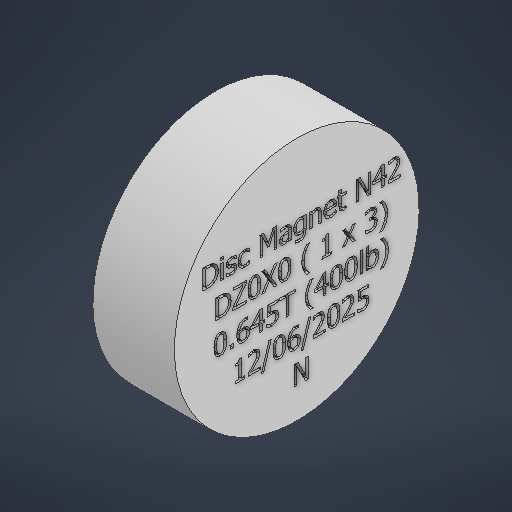
# Autodesk Inventor part: SampleMagnet
Saved by Autodesk Inventor 2026.1 (Build 301233000, 233)
## iProperties
Created: 2025-12-08
Part Number: SampleMagnet
Material: Generic
Document SubType Name: Modeling
Designer: usman
Density: 1 g/cm^3
Appearance: Default
Author: usman
Autodesk Inventor part; units mm, degrees
(part 1 of 2)
ref_plane "YZ Plane" through (0, 0, 0) normal (1, 0, 0) x (0, 1, 0)
ref_plane "XZ Plane" through (0, 0, 0) normal (0, 1, 0) x (-1, 0, 0)
ref_plane "XY Plane" through (0, 0, 0) normal (0, 0, 1) x (1, 0, 0)
sketch "Sketch1" plane through (0, 0, 0) normal (1, 0, 0) x (0, 1, 0)
  circle A0 centre (0, 0) radius 38.1
  dimension "d0" = 76.2
  constraints: 1 centre point, 1 coincident
  measures "d0" diameter of A0
extrude "Extrusion1" add sketch "Sketch1" along normal blind 25.4
sketch "Sketch2" plane through (25.4, 0, 0) normal (1, 0, 0) x (0, 0, -1)
  line L0 (-30.9138, 17.7652) -> (33.738, 17.7652) construction
  line L1 (33.738, 17.7652) -> (33.738, -46.1132) construction
  line L2 (33.738, -46.1132) -> (-30.9138, -46.1132) construction
  line L3 (-30.9138, -46.1132) -> (-30.9138, 17.7652) construction
  spline S0 degree 2 poles (-24.4539, 14.5839) (-24.4539, 13.749) (-25.1307, 12.4053) (-25.6988, 12.0299) knots 0 0 0 1 2 2 2
  spline S1 degree 2 poles (-25.6988, 12.0299) (-26.1632, 11.7384) (-27.1166, 11.5408) (-27.8576, 11.5408) knots 0 0 0 1 2 2 2
  line L4 (-27.8576, 11.5408) -> (-29.2606, 11.5408)
  line L5 (-29.2606, 11.5408) -> (-29.2606, 17.6368)
  line L6 (-29.2606, 17.6368) -> (-27.8724, 17.6368)
  spline S2 degree 2 poles (-27.8724, 17.6368) (-27.0129, 17.6368) (-26.0347, 17.3799) (-25.6889, 17.1527) knots 0 0 0 1 2 2 2
  spline S3 degree 2 poles (-25.6889, 17.1527) (-25.1011, 16.7624) (-24.4539, 15.4731) (-24.4539, 14.5839) knots 0 0 0 1 2 2 2
  spline S4 degree 2 poles (-25.2987, 14.5937) (-25.2987, 15.2952) (-25.763, 16.2882) (-26.2225, 16.5698) knots 0 0 0 1 2 2 2
  spline S5 degree 2 poles (-26.2225, 16.5698) (-26.5485, 16.7624) (-27.2846, 16.9353) (-27.8329, 16.9353) knots 0 0 0 1 2 2 2
  line L7 (-27.8329, 16.9353) -> (-28.4504, 16.9353)
  line L8 (-28.4504, 16.9353) -> (-28.4504, 12.2423)
  line L9 (-28.4504, 12.2423) -> (-27.8329, 12.2423)
  spline S6 degree 2 poles (-27.8329, 12.2423) (-27.2945, 12.2423) (-26.4793, 12.4152) (-26.1484, 12.6474) knots 0 0 0 1 2 2 2
  spline S7 degree 2 poles (-26.1484, 12.6474) (-25.7235, 12.9339) (-25.2987, 13.8824) (-25.2987, 14.5937) knots 0 0 0 1 2 2 2
  line L10 (-22.8484, 11.5408) -> (-23.6191, 11.5408)
  line L11 (-23.6191, 11.5408) -> (-23.6191, 16.1153)
  line L12 (-23.6191, 16.1153) -> (-22.8484, 16.1153)
  line L13 (-22.8484, 16.1153) -> (-22.8484, 11.5408)
  line L14 (-22.7941, 16.876) -> (-23.6685, 16.876)
  line L15 (-23.6685, 16.876) -> (-23.6685, 17.6763)
  line L16 (-23.6685, 17.6763) -> (-22.7941, 17.6763)
  line L17 (-22.7941, 17.6763) -> (-22.7941, 16.876)
  spline S8 degree 2 poles (-20.4821, 11.4321) (-20.9416, 11.4321) (-21.7369, 11.6791) (-21.9987, 11.8174) knots 0 0 0 1 2 2 2
  line L18 (-21.9987, 11.8174) -> (-21.9987, 12.6819)
  line L19 (-21.9987, 12.6819) -> (-21.9592, 12.6819)
  spline S9 degree 2 poles (-21.9592, 12.6819) (-21.8604, 12.6029) (-21.5937, 12.4152) (-21.3714, 12.3114) knots 0 0 0 1 2 2 2
  spline S10 degree 2 poles (-21.3714, 12.3114) (-21.1787, 12.2176) (-20.7044, 12.0793) (-20.4525, 12.0793) knots 0 0 0 1 2 2 2
  spline S11 degree 2 poles (-20.4525, 12.0793) (-20.2697, 12.0793) (-19.8498, 12.1632) (-19.751, 12.2324) knots 0 0 0 1 2 2 2
  spline S12 degree 2 poles (-19.751, 12.2324) (-19.6078, 12.3263) (-19.4793, 12.5387) (-19.4793, 12.756) knots 0 0 0 1 2 2 2
  spline S13 degree 2 poles (-19.4793, 12.756) (-19.4793, 13.0278) (-19.7757, 13.3093) (-20.1561, 13.4032) knots 0 0 0 1 2 2 2
  spline S14 degree 2 poles (-20.1561, 13.4032) (-20.3043, 13.4378) (-20.7786, 13.5366) (-20.9811, 13.5909) knots 0 0 0 1 2 2 2
  spline S15 degree 2 poles (-20.9811, 13.5909) (-21.5047, 13.7441) (-21.979, 14.3764) (-21.979, 14.8259) knots 0 0 0 1 2 2 2
  spline S16 degree 2 poles (-21.979, 14.8259) (-21.979, 15.4484) (-21.0453, 16.224) (-20.2747, 16.224) knots 0 0 0 1 2 2 2
  spline S17 degree 2 poles (-20.2747, 16.224) (-19.8943, 16.224) (-19.1236, 16.0362) (-18.8618, 15.893) knots 0 0 0 1 2 2 2
  line L20 (-18.8618, 15.893) -> (-18.8618, 15.068)
  line L21 (-18.8618, 15.068) -> (-18.9013, 15.068)
  spline S18 degree 2 poles (-18.9013, 15.068) (-19.1977, 15.3051) (-19.919, 15.5768) (-20.2895, 15.5768) knots 0 0 0 1 2 2 2
  spline S19 degree 2 poles (-20.2895, 15.5768) (-20.6699, 15.5768) (-21.1935, 15.2557) (-21.1935, 14.9346) knots 0 0 0 1 2 2 2
  spline S20 degree 2 poles (-21.1935, 14.9346) (-21.1935, 14.6431) (-20.8823, 14.3616) (-20.5365, 14.2726) knots 0 0 0 1 2 2 2
  spline S21 degree 2 poles (-20.5365, 14.2726) (-20.3685, 14.2282) (-19.9437, 14.1393) (-19.7115, 14.0849) knots 0 0 0 1 2 2 2
  spline S22 degree 2 poles (-19.7115, 14.0849) (-19.2076, 13.9565) (-18.6939, 13.3686) (-18.6939, 12.8598) knots 0 0 0 1 2 2 2
  spline S23 degree 2 poles (-18.6939, 12.8598) (-18.6939, 12.5634) (-18.926, 12.0397) (-19.1533, 11.8471) knots 0 0 0 1 2 2 2
  spline S24 degree 2 poles (-19.1533, 11.8471) (-19.3953, 11.6445) (-20.0128, 11.4321) (-20.4821, 11.4321) knots 0 0 0 1 2 2 2
  spline S25 degree 2 poles (-16.1596, 11.4371) (-16.6339, 11.4371) (-17.4193, 11.7285) (-17.7009, 12.0249) knots 0 0 0 1 2 2 2
  spline S26 degree 2 poles (-17.7009, 12.0249) (-17.9825, 12.3164) (-18.2937, 13.2155) (-18.2937, 13.8182) knots 0 0 0 1 2 2 2
  spline S27 degree 2 poles (-18.2937, 13.8182) (-18.2937, 14.4208) (-17.9726, 15.3002) (-17.7009, 15.5966) knots 0 0 0 1 2 2 2
  spline S28 degree 2 poles (-17.7009, 15.5966) (-17.4292, 15.8979) (-16.624, 16.219) (-16.1596, 16.219) knots 0 0 0 1 2 2 2
  spline S29 degree 2 poles (-16.1596, 16.219) (-15.7842, 16.219) (-15.0827, 16.0066) (-14.811, 15.8683) knots 0 0 0 1 2 2 2
  line L22 (-14.811, 15.8683) -> (-14.811, 15.0038)
  line L23 (-14.811, 15.0038) -> (-14.8555, 15.0038)
  spline S30 degree 2 poles (-14.8555, 15.0038) (-14.9394, 15.0729) (-15.1963, 15.2508) (-15.3791, 15.3446) knots 0 0 0 1 2 2 2
  spline S31 degree 2 poles (-15.3791, 15.3446) (-15.5421, 15.4237) (-15.9768, 15.5472) (-16.1744, 15.5472) knots 0 0 0 1 2 2 2
  spline S32 degree 2 poles (-16.1744, 15.5472) (-16.7722, 15.5472) (-17.4984, 14.6431) (-17.4984, 13.8182) knots 0 0 0 1 2 2 2
  spline S33 degree 2 poles (-17.4984, 13.8182) (-17.4984, 13.0129) (-16.7969, 12.1089) (-16.1744, 12.1089) knots 0 0 0 1 2 2 2
  spline S34 degree 2 poles (-16.1744, 12.1089) (-15.799, 12.1089) (-15.1173, 12.4201) (-14.8555, 12.6622) knots 0 0 0 1 2 2 2
  line L24 (-14.8555, 12.6622) -> (-14.811, 12.6622)
  line L25 (-14.811, 12.6622) -> (-14.811, 11.7977)
  spline S35 degree 2 poles (-14.811, 11.7977) (-14.9246, 11.7433) (-15.2704, 11.5902) (-15.4087, 11.5556) knots 0 0 0 1 2 2 2
  spline S36 degree 2 poles (-15.4087, 11.5556) (-15.6063, 11.4963) (-15.9176, 11.4371) (-16.1596, 11.4371) knots 0 0 0 1 2 2 2
  line L26 (-6.2055, 11.5408) -> (-7.0156, 11.5408)
  line L27 (-7.0156, 11.5408) -> (-7.0156, 16.7921)
  line L28 (-7.0156, 16.7921) -> (-8.6063, 13.2204)
  line L29 (-8.6063, 13.2204) -> (-9.1003, 13.2204)
  line L30 (-9.1003, 13.2204) -> (-10.6762, 16.7921)
  line L31 (-10.6762, 16.7921) -> (-10.6762, 11.5408)
  line L32 (-10.6762, 11.5408) -> (-11.432, 11.5408)
  line L33 (-11.432, 11.5408) -> (-11.432, 17.6368)
  line L34 (-11.432, 17.6368) -> (-10.3254, 17.6368)
  line L35 (-10.3254, 17.6368) -> (-8.8039, 14.243)
  line L36 (-8.8039, 14.243) -> (-7.3318, 17.6368)
  line L37 (-7.3318, 17.6368) -> (-6.2055, 17.6368)
  line L38 (-6.2055, 17.6368) -> (-6.2055, 11.5408)
  spline S37 degree 2 poles (-2.4807, 12.0249) (-2.5745, 11.9558) (-2.8907, 11.7088) (-3.0389, 11.6347) knots 0 0 0 1 2 2 2
  spline S38 degree 2 poles (-3.0389, 11.6347) (-3.2414, 11.526) (-3.6218, 11.4124) (-3.9676, 11.4124) knots 0 0 0 1 2 2 2
  spline S39 degree 2 poles (-3.9676, 11.4124) (-4.2492, 11.4124) (-4.758, 11.6248) (-4.9507, 11.8174) knots 0 0 0 1 2 2 2
  spline S40 degree 2 poles (-4.9507, 11.8174) (-5.1335, 12.0052) (-5.3558, 12.5584) (-5.3558, 12.8647) knots 0 0 0 1 2 2 2
  spline S41 degree 2 poles (-5.3558, 12.8647) (-5.3558, 13.339) (-4.9556, 14.0108) (-4.5209, 14.2035) knots 0 0 0 1 2 2 2
  spline S42 degree 2 poles (-4.5209, 14.2035) (-4.1356, 14.3813) (-3.0883, 14.5147) (-2.4807, 14.5493) knots 0 0 0 1 2 2 2
  line L39 (-2.4807, 14.5493) -> (-2.4807, 14.6975)
  spline S43 degree 2 poles (-2.4807, 14.6975) (-2.4807, 14.9642) (-2.6437, 15.2952) (-2.7919, 15.3891) knots 0 0 0 1 2 2 2
  spline S44 degree 2 poles (-2.7919, 15.3891) (-2.9401, 15.4829) (-3.3649, 15.5422) (-3.5922, 15.5422) knots 0 0 0 1 2 2 2
  spline S45 degree 2 poles (-3.5922, 15.5422) (-3.8589, 15.5422) (-4.5802, 15.3841) (-4.9408, 15.231) knots 0 0 0 1 2 2 2
  line L40 (-4.9408, 15.231) -> (-4.9853, 15.231)
  line L41 (-4.9853, 15.231) -> (-4.9853, 16.0165)
  spline S46 degree 2 poles (-4.9853, 16.0165) (-4.7728, 16.0758) (-3.9775, 16.224) (-3.5872, 16.224) knots 0 0 0 1 2 2 2
  spline S47 degree 2 poles (-3.5872, 16.224) (-3.113, 16.224) (-2.4658, 16.0758) (-2.209, 15.8831) knots 0 0 0 1 2 2 2
  spline S48 degree 2 poles (-2.209, 15.8831) (-1.957, 15.6954) (-1.71, 15.0976) (-1.71, 14.6678) knots 0 0 0 1 2 2 2
  line L42 (-1.71, 14.6678) -> (-1.71, 11.5408)
  line L43 (-1.71, 11.5408) -> (-2.4807, 11.5408)
  line L44 (-2.4807, 11.5408) -> (-2.4807, 12.0249)
  line L45 (-2.4807, 12.6671) -> (-2.4807, 13.9367)
  spline S49 degree 2 poles (-2.4807, 13.9367) (-2.7573, 13.912) (-3.5922, 13.828) (-3.854, 13.749) knots 0 0 0 1 2 2 2
  spline S50 degree 2 poles (-3.854, 13.749) (-4.1603, 13.6551) (-4.5604, 13.2649) (-4.5604, 12.9191) knots 0 0 0 1 2 2 2
  spline S51 degree 2 poles (-4.5604, 12.9191) (-4.5604, 12.5239) (-4.1158, 12.1237) (-3.691, 12.1237) knots 0 0 0 1 2 2 2
  spline S52 degree 2 poles (-3.691, 12.1237) (-3.3304, 12.1237) (-2.7376, 12.4349) (-2.4807, 12.6671) knots 0 0 0 1 2 2 2
  spline S53 degree 2 poles (-0.4651, 10.8097) (-0.3861, 10.7751) (-0.0848, 10.6664) (0.1079, 10.622) knots 0 0 0 1 2 2 2
  spline S54 degree 2 poles (0.1079, 10.622) (0.3203, 10.5676) (0.681, 10.5034) (0.8934, 10.5034) knots 0 0 0 1 2 2 2
  spline S55 degree 2 poles (0.8934, 10.5034) (1.2491, 10.5034) (1.7431, 10.6911) (1.8814, 10.8591) knots 0 0 0 1 2 2 2
  spline S56 degree 2 poles (1.8814, 10.8591) (2.0148, 11.027) (2.1185, 11.4667) (2.1185, 11.7483) knots 0 0 0 1 2 2 2
  line L46 (2.1185, 11.7483) -> (2.1185, 12.1484)
  spline S57 degree 2 poles (2.1185, 12.1484) (1.8073, 11.8767) (1.2095, 11.6198) (0.76, 11.6198) knots 0 0 0 1 2 2 2
  spline S58 degree 2 poles (0.76, 11.6198) (-0.0205, 11.6198) (-0.9443, 12.7807) (-0.9443, 13.8725) knots 0 0 0 1 2 2 2
  spline S59 degree 2 poles (-0.9443, 13.8725) (-0.9443, 14.4406) (-0.6232, 15.3199) (-0.3565, 15.6311) knots 0 0 0 1 2 2 2
  spline S60 degree 2 poles (-0.3565, 15.6311) (-0.0996, 15.9226) (0.6069, 16.2437) (0.9823, 16.2437) knots 0 0 0 1 2 2 2
  spline S61 degree 2 poles (0.9823, 16.2437) (1.338, 16.2437) (1.8567, 16.0758) (2.1185, 15.9226) knots 0 0 0 1 2 2 2
  line L47 (2.1185, 15.9226) -> (2.163, 16.1153)
  line L48 (2.163, 16.1153) -> (2.8891, 16.1153)
  line L49 (2.8891, 16.1153) -> (2.8891, 12.0644)
  spline S62 degree 2 poles (2.8891, 12.0644) (2.8891, 10.8986) (1.8764, 9.8118) (0.8341, 9.8118) knots 0 0 0 1 2 2 2
  spline S63 degree 2 poles (0.8341, 9.8118) (0.4982, 9.8118) (-0.2033, 9.9205) (-0.5047, 10.0094) knots 0 0 0 1 2 2 2
  line L50 (-0.5047, 10.0094) -> (-0.5047, 10.8097)
  line L51 (-0.5047, 10.8097) -> (-0.4651, 10.8097)
  line L52 (2.1185, 12.7807) -> (2.1185, 15.2952)
  spline S64 degree 2 poles (2.1185, 15.2952) (1.832, 15.4335) (1.3479, 15.5521) (1.1058, 15.5521) knots 0 0 0 1 2 2 2
  spline S65 degree 2 poles (1.1058, 15.5521) (0.5229, 15.5521) (-0.149, 14.6925) (-0.149, 13.8873) knots 0 0 0 1 2 2 2
  spline S66 degree 2 poles (-0.149, 13.8873) (-0.149, 13.1266) (0.3598, 12.3312) (0.9329, 12.3312) knots 0 0 0 1 2 2 2
  spline S67 degree 2 poles (0.9329, 12.3312) (1.2342, 12.3312) (1.8666, 12.5683) (2.1185, 12.7807) knots 0 0 0 1 2 2 2
  line L53 (7.597, 11.5408) -> (6.8264, 11.5408)
  line L54 (6.8264, 11.5408) -> (6.8264, 14.1491)
  spline S68 degree 2 poles (6.8264, 14.1491) (6.8264, 14.4653) (6.7671, 15.0087) (6.6782, 15.1717) knots 0 0 0 1 2 2 2
  spline S69 degree 2 poles (6.6782, 15.1717) (6.5843, 15.3446) (6.2484, 15.5126) (5.9618, 15.5126) knots 0 0 0 1 2 2 2
  spline S70 degree 2 poles (5.9618, 15.5126) (5.6753, 15.5126) (5.0677, 15.2063) (4.7762, 14.9593) knots 0 0 0 1 2 2 2
  line L55 (4.7762, 14.9593) -> (4.7762, 11.5408)
  line L56 (4.7762, 11.5408) -> (4.0056, 11.5408)
  line L57 (4.0056, 11.5408) -> (4.0056, 16.1153)
  line L58 (4.0056, 16.1153) -> (4.7762, 16.1153)
  line L59 (4.7762, 16.1153) -> (4.7762, 15.6064)
  spline S71 degree 2 poles (4.7762, 15.6064) (5.122, 15.9177) (5.7889, 16.2437) (6.1644, 16.2437) knots 0 0 0 1 2 2 2
  spline S72 degree 2 poles (6.1644, 16.2437) (6.8362, 16.2437) (7.597, 15.3545) (7.597, 14.5098) knots 0 0 0 1 2 2 2
  line L60 (7.597, 14.5098) -> (7.597, 11.5408)
  spline S73 degree 2 poles (10.6648, 11.4371) (9.5681, 11.4371) (8.3627, 12.6671) (8.3627, 13.8033) knots 0 0 0 1 2 2 2
  spline S74 degree 2 poles (8.3627, 13.8033) (8.3627, 14.9198) (9.5335, 16.2437) (10.477, 16.2437) knots 0 0 0 1 2 2 2
  spline S75 degree 2 poles (10.477, 16.2437) (10.9019, 16.2437) (11.5589, 15.9967) (11.801, 15.7349) knots 0 0 0 1 2 2 2
  spline S76 degree 2 poles (11.801, 15.7349) (12.048, 15.4731) (12.3098, 14.7172) (12.3098, 14.1689) knots 0 0 0 1 2 2 2
  line L61 (12.3098, 14.1689) -> (12.3098, 13.749)
  line L62 (12.3098, 13.749) -> (9.1432, 13.749)
  spline S77 degree 2 poles (9.1432, 13.749) (9.1432, 12.9537) (9.9435, 12.1089) (10.6549, 12.1089) knots 0 0 0 1 2 2 2
  spline S78 degree 2 poles (10.6549, 12.1089) (10.9068, 12.1089) (11.3959, 12.2225) (11.5935, 12.3114) knots 0 0 0 1 2 2 2
  spline S79 degree 2 poles (11.5935, 12.3114) (11.801, 12.4102) (12.0875, 12.5831) (12.1813, 12.6622) knots 0 0 0 1 2 2 2
  line L63 (12.1813, 12.6622) -> (12.2258, 12.6622)
  line L64 (12.2258, 12.6622) -> (12.2258, 11.8224)
  spline S80 degree 2 poles (12.2258, 11.8224) (12.0924, 11.768) (11.6873, 11.61) (11.5293, 11.5655) knots 0 0 0 1 2 2 2
  spline S81 degree 2 poles (11.5293, 11.5655) (11.307, 11.5013) (10.9414, 11.4371) (10.6648, 11.4371) knots 0 0 0 1 2 2 2
  spline S82 degree 2 poles (11.5589, 14.3369) (11.549, 14.6481) (11.4206, 15.1026) (11.2971, 15.2557) knots 0 0 0 1 2 2 2
  spline S83 degree 2 poles (11.2971, 15.2557) (11.1637, 15.4286) (10.7438, 15.6114) (10.4326, 15.6114) knots 0 0 0 1 2 2 2
  spline S84 degree 2 poles (10.4326, 15.6114) (10.1263, 15.6114) (9.6965, 15.4286) (9.5187, 15.2508) knots 0 0 0 1 2 2 2
  spline S85 degree 2 poles (9.5187, 15.2508) (9.3458, 15.068) (9.1679, 14.6283) (9.1432, 14.3369) knots 0 0 0 1 2 2 2
  line L65 (9.1432, 14.3369) -> (11.5589, 14.3369)
  spline S86 degree 2 poles (14.4735, 11.4519) (13.8461, 11.4519) (13.1397, 12.1682) (13.1397, 12.9438) knots 0 0 0 1 2 2 2
  line L66 (13.1397, 12.9438) -> (13.1397, 15.478)
  line L67 (13.1397, 15.478) -> (12.621, 15.478)
  line L68 (12.621, 15.478) -> (12.621, 16.1153)
  line L69 (12.621, 16.1153) -> (13.1397, 16.1153)
  line L70 (13.1397, 16.1153) -> (13.1397, 17.4293)
  line L71 (13.1397, 17.4293) -> (13.9104, 17.4293)
  line L72 (13.9104, 17.4293) -> (13.9104, 16.1153)
  line L73 (13.9104, 16.1153) -> (15.3281, 16.1153)
  line L74 (15.3281, 16.1153) -> (15.3281, 15.478)
  line L75 (15.3281, 15.478) -> (13.9104, 15.478)
  line L76 (13.9104, 15.478) -> (13.9104, 13.2995)
  spline S87 degree 2 poles (13.9104, 13.2995) (13.9104, 12.9537) (13.9351, 12.5733) (14.019, 12.4102) knots 0 0 0 1 2 2 2
  spline S88 degree 2 poles (14.019, 12.4102) (14.0882, 12.267) (14.3994, 12.1237) (14.6662, 12.1237) knots 0 0 0 1 2 2 2
  spline S89 degree 2 poles (14.6662, 12.1237) (14.8539, 12.1237) (15.2046, 12.2373) (15.2837, 12.2719) knots 0 0 0 1 2 2 2
  line L77 (15.2837, 12.2719) -> (15.3281, 12.2719)
  line L78 (15.3281, 12.2719) -> (15.3281, 11.5803)
  spline S90 degree 2 poles (15.3281, 11.5803) (15.1108, 11.521) (14.6662, 11.4519) (14.4735, 11.4519) knots 0 0 0 1 2 2 2
  line L79 (22.9358, 11.5408) -> (22.0268, 11.5408)
  line L80 (22.0268, 11.5408) -> (19.3296, 16.797)
  line L81 (19.3296, 16.797) -> (19.3296, 11.5408)
  line L82 (19.3296, 11.5408) -> (18.5737, 11.5408)
  line L83 (18.5737, 11.5408) -> (18.5737, 17.6368)
  line L84 (18.5737, 17.6368) -> (19.7248, 17.6368)
  line L85 (19.7248, 17.6368) -> (22.18, 12.8104)
  line L86 (22.18, 12.8104) -> (22.18, 17.6368)
  line L87 (22.18, 17.6368) -> (22.9358, 17.6368)
  line L88 (22.9358, 17.6368) -> (22.9358, 11.5408)
  line L89 (27.9203, 13.6354) -> (27.1941, 13.6354)
  line L90 (27.1941, 13.6354) -> (27.1941, 11.5408)
  line L91 (27.1941, 11.5408) -> (26.4086, 11.5408)
  line L92 (26.4086, 11.5408) -> (26.4086, 13.6354)
  line L93 (26.4086, 13.6354) -> (23.7163, 13.6354)
  line L94 (23.7163, 13.6354) -> (23.7163, 14.4949)
  line L95 (23.7163, 14.4949) -> (26.4432, 17.6368)
  line L96 (26.4432, 17.6368) -> (27.1941, 17.6368)
  line L97 (27.1941, 17.6368) -> (27.1941, 14.2924)
  line L98 (27.1941, 14.2924) -> (27.9203, 14.2924)
  line L99 (27.9203, 14.2924) -> (27.9203, 13.6354)
  line L100 (26.4086, 14.2924) -> (26.4086, 16.6735)
  line L101 (26.4086, 16.6735) -> (24.3585, 14.2924)
  line L102 (24.3585, 14.2924) -> (26.4086, 14.2924)
  line L103 (32.3317, 11.5408) -> (28.5724, 11.5408)
  line L104 (28.5724, 11.5408) -> (28.5724, 12.4053)
  spline S91 degree 2 poles (28.5724, 12.4053) (28.9775, 12.7857) (29.6987, 13.4921) (30.0445, 13.8725) knots 0 0 0 1 2 2 2
  spline S92 degree 2 poles (30.0445, 13.8725) (30.741, 14.6382) (31.2499, 15.557) (31.2499, 16.0461) knots 0 0 0 1 2 2 2
  spline S93 degree 2 poles (31.2499, 16.0461) (31.2499, 16.303) (31.0918, 16.6883) (30.9485, 16.8118) knots 0 0 0 1 2 2 2
  spline S94 degree 2 poles (30.9485, 16.8118) (30.8053, 16.9353) (30.4298, 17.0588) (30.2026, 17.0588) knots 0 0 0 1 2 2 2
  spline S95 degree 2 poles (30.2026, 17.0588) (29.9852, 17.0588) (29.5406, 16.9501) (29.3381, 16.8662) knots 0 0 0 1 2 2 2
  spline S96 degree 2 poles (29.3381, 16.8662) (29.1652, 16.797) (28.8441, 16.5994) (28.7453, 16.5302) knots 0 0 0 1 2 2 2
  line L105 (28.7453, 16.5302) -> (28.7008, 16.5302)
  line L106 (28.7008, 16.5302) -> (28.7008, 17.3997)
  spline S97 degree 2 poles (28.7008, 17.3997) (28.9528, 17.5232) (29.8568, 17.7652) (30.2619, 17.7652) knots 0 0 0 1 2 2 2
  spline S98 degree 2 poles (30.2619, 17.7652) (31.1165, 17.7652) (32.0798, 16.8612) (32.0798, 16.0906) knots 0 0 0 1 2 2 2
  spline S99 degree 2 poles (32.0798, 16.0906) (32.0798, 15.7299) (31.9118, 15.1273) (31.7636, 14.8704) knots 0 0 0 1 2 2 2
  spline S100 degree 2 poles (31.7636, 14.8704) (31.6154, 14.6036) (31.1857, 14.08) (30.9485, 13.828) knots 0 0 0 1 2 2 2
  spline S101 degree 2 poles (30.9485, 13.828) (30.5632, 13.4081) (29.6197, 12.509) (29.3381, 12.2472) knots 0 0 0 1 2 2 2
  line L107 (29.3381, 12.2472) -> (32.3317, 12.2472)
  line L108 (32.3317, 12.2472) -> (32.3317, 11.5408)
  spline S102 degree 2 poles (-20.455, 4.547) (-20.455, 3.7121) (-21.1318, 2.3684) (-21.6999, 1.993) knots 0 0 0 1 2 2 2
  spline S103 degree 2 poles (-21.6999, 1.993) (-22.1642, 1.7015) (-23.1177, 1.5039) (-23.8587, 1.5039) knots 0 0 0 1 2 2 2
  line L109 (-23.8587, 1.5039) -> (-25.2616, 1.5039)
  line L110 (-25.2616, 1.5039) -> (-25.2616, 7.5999)
  line L111 (-25.2616, 7.5999) -> (-23.8735, 7.5999)
  spline S104 degree 2 poles (-23.8735, 7.5999) (-23.0139, 7.5999) (-22.0358, 7.343) (-21.69, 7.1158) knots 0 0 0 1 2 2 2
  spline S105 degree 2 poles (-21.69, 7.1158) (-21.1021, 6.7255) (-20.455, 5.4362) (-20.455, 4.547) knots 0 0 0 1 2 2 2
  spline S106 degree 2 poles (-21.2997, 4.5568) (-21.2997, 5.2583) (-21.7641, 6.2513) (-22.2235, 6.5329) knots 0 0 0 1 2 2 2
  spline S107 degree 2 poles (-22.2235, 6.5329) (-22.5496, 6.7255) (-23.2856, 6.8984) (-23.834, 6.8984) knots 0 0 0 1 2 2 2
  line L112 (-23.834, 6.8984) -> (-24.4515, 6.8984)
  line L113 (-24.4515, 6.8984) -> (-24.4515, 2.2054)
  line L114 (-24.4515, 2.2054) -> (-23.834, 2.2054)
  spline S108 degree 2 poles (-23.834, 2.2054) (-23.2955, 2.2054) (-22.4804, 2.3783) (-22.1494, 2.6105) knots 0 0 0 1 2 2 2
  spline S109 degree 2 poles (-22.1494, 2.6105) (-21.7246, 2.897) (-21.2997, 3.8455) (-21.2997, 4.5568) knots 0 0 0 1 2 2 2
  line L115 (-15.6878, 1.5039) -> (-19.9462, 1.5039)
  line L116 (-19.9462, 1.5039) -> (-19.9462, 2.2597)
  line L117 (-19.9462, 2.2597) -> (-16.6857, 6.8787)
  line L118 (-16.6857, 6.8787) -> (-19.798, 6.8787)
  line L119 (-19.798, 6.8787) -> (-19.798, 7.5999)
  line L120 (-19.798, 7.5999) -> (-15.7718, 7.5999)
  line L121 (-15.7718, 7.5999) -> (-15.7718, 6.8688)
  line L122 (-15.7718, 6.8688) -> (-19.0668, 2.2251)
  line L123 (-19.0668, 2.2251) -> (-15.6878, 2.2251)
  line L124 (-15.6878, 2.2251) -> (-15.6878, 1.5039)
  spline S110 degree 2 poles (-11.2665, 4.5519) (-11.2665, 2.9118) (-12.2199, 1.3755) (-13.2129, 1.3755) knots 0 0 0 1 2 2 2
  spline S111 degree 2 poles (-13.2129, 1.3755) (-14.2207, 1.3755) (-15.1642, 2.9414) (-15.1642, 4.547) knots 0 0 0 1 2 2 2
  spline S112 degree 2 poles (-15.1642, 4.547) (-15.1642, 6.1969) (-14.2108, 7.7234) (-13.2129, 7.7234) knots 0 0 0 1 2 2 2
  spline S113 degree 2 poles (-13.2129, 7.7234) (-12.2101, 7.7234) (-11.2665, 6.1426) (-11.2665, 4.5519) knots 0 0 0 1 2 2 2
  spline S114 degree 2 poles (-12.3138, 2.6944) (-12.1952, 2.9958) (-12.0964, 3.9245) (-12.0964, 4.5519) knots 0 0 0 1 2 2 2
  spline S115 degree 2 poles (-12.0964, 4.5519) (-12.0964, 5.1793) (-12.1952, 6.1031) (-12.3187, 6.4143) knots 0 0 0 1 2 2 2
  spline S116 degree 2 poles (-12.3187, 6.4143) (-12.4422, 6.7255) (-12.872, 7.0466) (-13.2129, 7.0466) knots 0 0 0 1 2 2 2
  spline S117 degree 2 poles (-13.2129, 7.0466) (-13.5538, 7.0466) (-13.9934, 6.7255) (-14.1219, 6.4044) knots 0 0 0 1 2 2 2
  spline S118 degree 2 poles (-14.1219, 6.4044) (-14.2454, 6.0932) (-14.3343, 5.1447) (-14.3343, 4.547) knots 0 0 0 1 2 2 2
  spline S119 degree 2 poles (-14.3343, 4.547) (-14.3343, 3.9048) (-14.2552, 3.0452) (-14.1268, 2.7093) knots 0 0 0 1 2 2 2
  spline S120 degree 2 poles (-14.1268, 2.7093) (-14.0082, 2.3931) (-13.5686, 2.0522) (-13.2129, 2.0522) knots 0 0 0 1 2 2 2
  spline S121 degree 2 poles (-13.2129, 2.0522) (-12.877, 2.0522) (-12.4373, 2.3733) (-12.3138, 2.6944) knots 0 0 0 1 2 2 2
  line L125 (-6.0992, 1.5039) -> (-7.028, 1.5039)
  line L126 (-7.028, 1.5039) -> (-8.51, 3.9344)
  line L127 (-8.51, 3.9344) -> (-10.0216, 1.5039)
  line L128 (-10.0216, 1.5039) -> (-10.896, 1.5039)
  line L129 (-10.896, 1.5039) -> (-8.9546, 4.5568)
  line L130 (-8.9546, 4.5568) -> (-10.8367, 7.5999)
  line L131 (-10.8367, 7.5999) -> (-9.908, 7.5999)
  line L132 (-9.908, 7.5999) -> (-8.4556, 5.2139)
  line L133 (-8.4556, 5.2139) -> (-6.9736, 7.5999)
  line L134 (-6.9736, 7.5999) -> (-6.0992, 7.5999)
  line L135 (-6.0992, 7.5999) -> (-8.0061, 4.5964)
  line L136 (-8.0061, 4.5964) -> (-6.0992, 1.5039)
  spline S122 degree 2 poles (-1.8261, 4.5519) (-1.8261, 2.9118) (-2.7795, 1.3755) (-3.7725, 1.3755) knots 0 0 0 1 2 2 2
  spline S123 degree 2 poles (-3.7725, 1.3755) (-4.7803, 1.3755) (-5.7238, 2.9414) (-5.7238, 4.547) knots 0 0 0 1 2 2 2
  spline S124 degree 2 poles (-5.7238, 4.547) (-5.7238, 6.1969) (-4.7704, 7.7234) (-3.7725, 7.7234) knots 0 0 0 1 2 2 2
  spline S125 degree 2 poles (-3.7725, 7.7234) (-2.7697, 7.7234) (-1.8261, 6.1426) (-1.8261, 4.5519) knots 0 0 0 1 2 2 2
  spline S126 degree 2 poles (-2.8734, 2.6944) (-2.7548, 2.9958) (-2.656, 3.9245) (-2.656, 4.5519) knots 0 0 0 1 2 2 2
  spline S127 degree 2 poles (-2.656, 4.5519) (-2.656, 5.1793) (-2.7548, 6.1031) (-2.8783, 6.4143) knots 0 0 0 1 2 2 2
  spline S128 degree 2 poles (-2.8783, 6.4143) (-3.0018, 6.7255) (-3.4316, 7.0466) (-3.7725, 7.0466) knots 0 0 0 1 2 2 2
  spline S129 degree 2 poles (-3.7725, 7.0466) (-4.1134, 7.0466) (-4.553, 6.7255) (-4.6815, 6.4044) knots 0 0 0 1 2 2 2
  spline S130 degree 2 poles (-4.6815, 6.4044) (-4.805, 6.0932) (-4.8939, 5.1447) (-4.8939, 4.547) knots 0 0 0 1 2 2 2
  spline S131 degree 2 poles (-4.8939, 4.547) (-4.8939, 3.9048) (-4.8148, 3.0452) (-4.6864, 2.7093) knots 0 0 0 1 2 2 2
  spline S132 degree 2 poles (-4.6864, 2.7093) (-4.5678, 2.3931) (-4.1282, 2.0522) (-3.7725, 2.0522) knots 0 0 0 1 2 2 2
  spline S133 degree 2 poles (-3.7725, 2.0522) (-3.4366, 2.0522) (-2.9969, 2.3733) (-2.8734, 2.6944) knots 0 0 0 1 2 2 2
  line L137 (4.0328, -0.1807) -> (3.0942, -0.1807)
  spline S134 degree 2 poles (3.0942, -0.1807) (2.3828, 0.6641) (1.5677, 2.5561) (1.5677, 3.8455) knots 0 0 0 1 2 2 2
  spline S135 degree 2 poles (1.5677, 3.8455) (1.5677, 5.1052) (2.3729, 7.0269) (3.0942, 7.8716) knots 0 0 0 1 2 2 2
  line L138 (3.0942, 7.8716) -> (4.0328, 7.8716)
  line L139 (4.0328, 7.8716) -> (4.0328, 7.8321)
  spline S136 degree 2 poles (4.0328, 7.8321) (3.7018, 7.5307) (3.0991, 6.7502) (2.8422, 6.2315) knots 0 0 0 1 2 2 2
  spline S137 degree 2 poles (2.8422, 6.2315) (2.5952, 5.7276) (2.2889, 4.5173) (2.2889, 3.8455) knots 0 0 0 1 2 2 2
  spline S138 degree 2 poles (2.2889, 3.8455) (2.2889, 3.144) (2.5853, 1.9831) (2.8422, 1.4594) knots 0 0 0 1 2 2 2
  spline S139 degree 2 poles (2.8422, 1.4594) (3.0892, 0.9556) (3.7166, 0.1404) (4.0328, -0.1411) knots 0 0 0 1 2 2 2
  line L140 (4.0328, -0.1411) -> (4.0328, -0.1807)
  line L141 (10.8549, 1.5039) -> (7.881, 1.5039)
  line L142 (7.881, 1.5039) -> (7.881, 2.1263)
  line L143 (7.881, 2.1263) -> (8.9876, 2.1263)
  line L144 (8.9876, 2.1263) -> (8.9876, 6.2117)
  line L145 (8.9876, 6.2117) -> (7.881, 6.2117)
  line L146 (7.881, 6.2117) -> (7.881, 6.77)
  spline S140 degree 2 poles (7.881, 6.77) (8.5084, 6.77) (9.1012, 7.1257) (9.1408, 7.6197) knots 0 0 0 1 2 2 2
  line L147 (9.1408, 7.6197) -> (9.7731, 7.6197)
  line L148 (9.7731, 7.6197) -> (9.7731, 2.1263)
  line L149 (9.7731, 2.1263) -> (10.8549, 2.1263)
  line L150 (10.8549, 2.1263) -> (10.8549, 1.5039)
  line L151 (18.2601, 1.5039) -> (17.3165, 1.5039)
  line L152 (17.3165, 1.5039) -> (16.205, 3.223)
  line L153 (16.205, 3.223) -> (15.0639, 1.5039)
  line L154 (15.0639, 1.5039) -> (14.1895, 1.5039)
  line L155 (14.1895, 1.5039) -> (15.7752, 3.7714)
  line L156 (15.7752, 3.7714) -> (14.2043, 6.0784)
  line L157 (14.2043, 6.0784) -> (15.1478, 6.0784)
  line L158 (15.1478, 6.0784) -> (16.2544, 4.3741)
  line L159 (16.2544, 4.3741) -> (17.3857, 6.0784)
  line L160 (17.3857, 6.0784) -> (18.2601, 6.0784)
  line L161 (18.2601, 6.0784) -> (16.6842, 3.8208)
  line L162 (16.6842, 3.8208) -> (18.2601, 1.5039)
  spline S141 degree 2 poles (23.0074, 7.0219) (22.7851, 7.0219) (22.3455, 6.9132) (22.133, 6.8293) knots 0 0 0 1 2 2 2
  spline S142 degree 2 poles (22.133, 6.8293) (21.9354, 6.7453) (21.644, 6.5674) (21.5304, 6.4884) knots 0 0 0 1 2 2 2
  line L163 (21.5304, 6.4884) -> (21.481, 6.4884)
  line L164 (21.481, 6.4884) -> (21.481, 7.3529)
  spline S143 degree 2 poles (21.481, 7.3529) (21.7477, 7.4962) (22.6616, 7.7283) (23.0716, 7.7283) knots 0 0 0 1 2 2 2
  spline S144 degree 2 poles (23.0716, 7.7283) (23.4866, 7.7283) (24.1041, 7.5604) (24.3561, 7.3825) knots 0 0 0 1 2 2 2
  spline S145 degree 2 poles (24.3561, 7.3825) (24.6228, 7.1899) (24.8995, 6.6317) (24.8995, 6.2562) knots 0 0 0 1 2 2 2
  spline S146 degree 2 poles (24.8995, 6.2562) (24.8995, 5.7523) (24.2375, 4.9916) (23.7731, 4.8928) knots 0 0 0 1 2 2 2
  line L165 (23.7731, 4.8928) -> (23.7731, 4.8335)
  spline S147 degree 2 poles (23.7731, 4.8335) (23.9658, 4.794) (24.4055, 4.6161) (24.5932, 4.4383) knots 0 0 0 1 2 2 2
  spline S148 degree 2 poles (24.5932, 4.4383) (24.7809, 4.2654) (25.018, 3.7121) (25.018, 3.3119) knots 0 0 0 1 2 2 2
  spline S149 degree 2 poles (25.018, 3.3119) (25.018, 2.9019) (24.7364, 2.2054) (24.4796, 1.9386) knots 0 0 0 1 2 2 2
  spline S150 degree 2 poles (24.4796, 1.9386) (24.2128, 1.662) (23.457, 1.3755) (22.9778, 1.3755) knots 0 0 0 1 2 2 2
  spline S151 degree 2 poles (22.9778, 1.3755) (22.5184, 1.3755) (21.6193, 1.5978) (21.313, 1.7509) knots 0 0 0 1 2 2 2
  line L166 (21.313, 1.7509) -> (21.313, 2.6154)
  line L167 (21.313, 2.6154) -> (21.3723, 2.6154)
  spline S152 degree 2 poles (21.3723, 2.6154) (21.6292, 2.4277) (22.4986, 2.0819) (22.9284, 2.0819) knots 0 0 0 1 2 2 2
  spline S153 degree 2 poles (22.9284, 2.0819) (23.1803, 2.0819) (23.6842, 2.24) (23.8522, 2.4227) knots 0 0 0 1 2 2 2
  spline S154 degree 2 poles (23.8522, 2.4227) (24.0152, 2.6055) (24.1881, 3.0402) (24.1881, 3.3712) knots 0 0 0 1 2 2 2
  spline S155 degree 2 poles (24.1881, 3.3712) (24.1881, 3.7022) (23.9954, 4.132) (23.8225, 4.2555) knots 0 0 0 1 2 2 2
  spline S156 degree 2 poles (23.8225, 4.2555) (23.6496, 4.379) (23.1803, 4.4729) (22.9037, 4.4729) knots 0 0 0 1 2 2 2
  line L168 (22.9037, 4.4729) -> (22.5579, 4.4729)
  line L169 (22.5579, 4.4729) -> (22.5579, 5.1496)
  line L170 (22.5579, 5.1496) -> (22.8296, 5.1496)
  spline S157 degree 2 poles (22.8296, 5.1496) (23.3779, 5.1496) (24.0695, 5.6733) (24.0695, 6.1722) knots 0 0 0 1 2 2 2
  spline S158 degree 2 poles (24.0695, 6.1722) (24.0695, 6.4044) (23.8917, 6.7354) (23.7484, 6.8342) knots 0 0 0 1 2 2 2
  spline S159 degree 2 poles (23.7484, 6.8342) (23.5953, 6.9379) (23.2198, 7.0219) (23.0074, 7.0219) knots 0 0 0 1 2 2 2
  spline S160 degree 2 poles (28.2636, 3.8455) (28.2636, 2.5808) (27.4535, 0.6641) (26.7372, -0.1807) knots 0 0 0 1 2 2 2
  line L171 (26.7372, -0.1807) -> (25.7985, -0.1807)
  line L172 (25.7985, -0.1807) -> (25.7985, -0.1411)
  spline S161 degree 2 poles (25.7985, -0.1411) (26.1147, 0.1404) (26.752, 0.9654) (26.9891, 1.4594) knots 0 0 0 1 2 2 2
  spline S162 degree 2 poles (26.9891, 1.4594) (27.246, 1.988) (27.5424, 3.1637) (27.5424, 3.8455) knots 0 0 0 1 2 2 2
  spline S163 degree 2 poles (27.5424, 3.8455) (27.5424, 4.5223) (27.241, 5.7227) (26.9891, 6.2315) knots 0 0 0 1 2 2 2
  spline S164 degree 2 poles (26.9891, 6.2315) (26.7421, 6.7403) (26.1098, 7.5505) (25.7985, 7.8321) knots 0 0 0 1 2 2 2
  line L173 (25.7985, 7.8321) -> (25.7985, 7.8716)
  line L174 (25.7985, 7.8716) -> (26.7372, 7.8716)
  spline S165 degree 2 poles (26.7372, 7.8716) (27.4485, 7.0269) (28.2636, 5.12) (28.2636, 3.8455) knots 0 0 0 1 2 2 2
  spline S166 degree 2 poles (-21.8728, -5.485) (-21.8728, -7.1251) (-22.8262, -8.6614) (-23.8191, -8.6614) knots 0 0 0 1 2 2 2
  spline S167 degree 2 poles (-23.8191, -8.6614) (-24.8269, -8.6614) (-25.7705, -7.0955) (-25.7705, -5.4899) knots 0 0 0 1 2 2 2
  spline S168 degree 2 poles (-25.7705, -5.4899) (-25.7705, -3.84) (-24.817, -2.3135) (-23.8191, -2.3135) knots 0 0 0 1 2 2 2
  spline S169 degree 2 poles (-23.8191, -2.3135) (-22.8163, -2.3135) (-21.8728, -3.8943) (-21.8728, -5.485) knots 0 0 0 1 2 2 2
  spline S170 degree 2 poles (-22.9201, -7.3425) (-22.8015, -7.0411) (-22.7027, -6.1124) (-22.7027, -5.485) knots 0 0 0 1 2 2 2
  spline S171 degree 2 poles (-22.7027, -5.485) (-22.7027, -4.8576) (-22.8015, -3.9338) (-22.925, -3.6226) knots 0 0 0 1 2 2 2
  spline S172 degree 2 poles (-22.925, -3.6226) (-23.0485, -3.3114) (-23.4783, -2.9903) (-23.8191, -2.9903) knots 0 0 0 1 2 2 2
  spline S173 degree 2 poles (-23.8191, -2.9903) (-24.16, -2.9903) (-24.5997, -3.3114) (-24.7281, -3.6325) knots 0 0 0 1 2 2 2
  spline S174 degree 2 poles (-24.7281, -3.6325) (-24.8516, -3.9437) (-24.9405, -4.8922) (-24.9405, -5.4899) knots 0 0 0 1 2 2 2
  spline S175 degree 2 poles (-24.9405, -5.4899) (-24.9405, -6.1321) (-24.8615, -6.9917) (-24.733, -7.3276) knots 0 0 0 1 2 2 2
  spline S176 degree 2 poles (-24.733, -7.3276) (-24.6145, -7.6438) (-24.1748, -7.9847) (-23.8191, -7.9847) knots 0 0 0 1 2 2 2
  spline S177 degree 2 poles (-23.8191, -7.9847) (-23.4832, -7.9847) (-23.0436, -7.6636) (-22.9201, -7.3425) knots 0 0 0 1 2 2 2
  line L175 (-19.7831, -8.533) -> (-20.7613, -8.533)
  line L176 (-20.7613, -8.533) -> (-20.7613, -7.3672)
  line L177 (-20.7613, -7.3672) -> (-19.7831, -7.3672)
  line L178 (-19.7831, -7.3672) -> (-19.7831, -8.533)
  spline S178 degree 2 poles (-14.6998, -6.557) (-14.6998, -7.0263) (-15.0111, -7.8216) (-15.2729, -8.0884) knots 0 0 0 1 2 2 2
  spline S179 degree 2 poles (-15.2729, -8.0884) (-15.5446, -8.37) (-16.2263, -8.6614) (-16.6363, -8.6614) knots 0 0 0 1 2 2 2
  spline S180 degree 2 poles (-16.6363, -8.6614) (-17.0464, -8.6614) (-17.7231, -8.3848) (-17.98, -8.1082) knots 0 0 0 1 2 2 2
  spline S181 degree 2 poles (-17.98, -8.1082) (-18.2962, -7.7772) (-18.6519, -6.6657) (-18.6519, -5.8555) knots 0 0 0 1 2 2 2
  spline S182 degree 2 poles (-18.6519, -5.8555) (-18.6519, -5.0602) (-18.3258, -3.7807) (-17.985, -3.3065) knots 0 0 0 1 2 2 2
  spline S183 degree 2 poles (-17.985, -3.3065) (-17.654, -2.8421) (-16.6067, -2.3234) (-15.92, -2.3234) knots 0 0 0 1 2 2 2
  spline S184 degree 2 poles (-15.92, -2.3234) (-15.7175, -2.3234) (-15.3618, -2.3629) (-15.2284, -2.4074) knots 0 0 0 1 2 2 2
  line L179 (-15.2284, -2.4074) -> (-15.2284, -3.1928)
  line L180 (-15.2284, -3.1928) -> (-15.263, -3.1928)
  spline S185 degree 2 poles (-15.263, -3.1928) (-15.3766, -3.1336) (-15.7916, -3.0298) (-16.0287, -3.0298) knots 0 0 0 1 2 2 2
  spline S186 degree 2 poles (-16.0287, -3.0298) (-16.7895, -3.0298) (-17.7231, -4.0573) (-17.8121, -5.0651) knots 0 0 0 1 2 2 2
  spline S187 degree 2 poles (-17.8121, -5.0651) (-17.5206, -4.8626) (-16.908, -4.6403) (-16.5425, -4.6403) knots 0 0 0 1 2 2 2
  spline S188 degree 2 poles (-16.5425, -4.6403) (-16.1868, -4.6403) (-15.6533, -4.7835) (-15.3618, -5.0009) knots 0 0 0 1 2 2 2
  spline S189 degree 2 poles (-15.3618, -5.0009) (-15.0259, -5.2528) (-14.6998, -6.0333) (-14.6998, -6.557) knots 0 0 0 1 2 2 2
  spline S190 degree 2 poles (-15.5298, -6.5916) (-15.5298, -6.2161) (-15.7274, -5.7073) (-15.9447, -5.5295) knots 0 0 0 1 2 2 2
  spline S191 degree 2 poles (-15.9447, -5.5295) (-16.1078, -5.401) (-16.5128, -5.317) (-16.7253, -5.317) knots 0 0 0 1 2 2 2
  spline S192 degree 2 poles (-16.7253, -5.317) (-17.0118, -5.317) (-17.5502, -5.4899) (-17.8121, -5.653) knots 0 0 0 1 2 2 2
  spline S193 degree 2 poles (-17.8121, -5.653) (-17.817, -5.7419) (-17.8269, -5.9098) (-17.8269, -6.0383) knots 0 0 0 1 2 2 2
  spline S194 degree 2 poles (-17.8269, -6.0383) (-17.8269, -6.6706) (-17.5799, -7.4462) (-17.3922, -7.6487) knots 0 0 0 1 2 2 2
  spline S195 degree 2 poles (-17.3922, -7.6487) (-17.2193, -7.8414) (-16.8438, -7.9945) (-16.6314, -7.9945) knots 0 0 0 1 2 2 2
  spline S196 degree 2 poles (-16.6314, -7.9945) (-16.1374, -7.9945) (-15.5298, -7.2931) (-15.5298, -6.5916) knots 0 0 0 1 2 2 2
  line L181 (-10.0562, -6.4384) -> (-10.7824, -6.4384)
  line L182 (-10.7824, -6.4384) -> (-10.7824, -8.533)
  line L183 (-10.7824, -8.533) -> (-11.5679, -8.533)
  line L184 (-11.5679, -8.533) -> (-11.5679, -6.4384)
  line L185 (-11.5679, -6.4384) -> (-14.2602, -6.4384)
  line L186 (-14.2602, -6.4384) -> (-14.2602, -5.5789)
  line L187 (-14.2602, -5.5789) -> (-11.5333, -2.437)
  line L188 (-11.5333, -2.437) -> (-10.7824, -2.437)
  line L189 (-10.7824, -2.437) -> (-10.7824, -5.7814)
  line L190 (-10.7824, -5.7814) -> (-10.0562, -5.7814)
  line L191 (-10.0562, -5.7814) -> (-10.0562, -6.4384)
  line L192 (-11.5679, -5.7814) -> (-11.5679, -3.4003)
  line L193 (-11.5679, -3.4003) -> (-13.618, -5.7814)
  line L194 (-13.618, -5.7814) -> (-11.5679, -5.7814)
  spline S197 degree 2 poles (-5.709, -6.5965) (-5.709, -7.0362) (-5.9906, -7.7871) (-6.2474, -8.0637) knots 0 0 0 1 2 2 2
  spline S198 degree 2 poles (-6.2474, -8.0637) (-6.5043, -8.3403) (-7.27, -8.6614) (-7.7443, -8.6614) knots 0 0 0 1 2 2 2
  spline S199 degree 2 poles (-7.7443, -8.6614) (-8.179, -8.6614) (-9.0287, -8.4688) (-9.3399, -8.3156) knots 0 0 0 1 2 2 2
  line L195 (-9.3399, -8.3156) -> (-9.3399, -7.4511)
  line L196 (-9.3399, -7.4511) -> (-9.2806, -7.4511)
  spline S200 degree 2 poles (-9.2806, -7.4511) (-9.1868, -7.5203) (-8.836, -7.6981) (-8.6236, -7.7772) knots 0 0 0 1 2 2 2
  spline S201 degree 2 poles (-8.6236, -7.7772) (-8.3815, -7.8612) (-7.9814, -7.955) (-7.7295, -7.955) knots 0 0 0 1 2 2 2
  spline S202 degree 2 poles (-7.7295, -7.955) (-7.4825, -7.955) (-7.0181, -7.7772) (-6.8501, -7.5845) knots 0 0 0 1 2 2 2
  spline S203 degree 2 poles (-6.8501, -7.5845) (-6.697, -7.4017) (-6.5389, -6.9176) (-6.5389, -6.5916) knots 0 0 0 1 2 2 2
  spline S204 degree 2 poles (-6.5389, -6.5916) (-6.5389, -6.2655) (-6.7167, -5.8506) (-6.8847, -5.7122) knots 0 0 0 1 2 2 2
  spline S205 degree 2 poles (-6.8847, -5.7122) (-7.0576, -5.5591) (-7.5714, -5.4307) (-7.8826, -5.4307) knots 0 0 0 1 2 2 2
  spline S206 degree 2 poles (-7.8826, -5.4307) (-8.2185, -5.4307) (-8.8854, -5.5344) (-9.088, -5.5789) knots 0 0 0 1 2 2 2
  line L197 (-9.088, -5.5789) -> (-9.088, -2.437)
  line L198 (-9.088, -2.437) -> (-5.7436, -2.437)
  line L199 (-5.7436, -2.437) -> (-5.7436, -3.1533)
  line L200 (-5.7436, -3.1533) -> (-8.3025, -3.1533)
  line L201 (-8.3025, -3.1533) -> (-8.3025, -4.7786)
  spline S207 degree 2 poles (-8.3025, -4.7786) (-8.1543, -4.7588) (-7.8678, -4.744) (-7.7492, -4.744) knots 0 0 0 1 2 2 2
  spline S208 degree 2 poles (-7.7492, -4.744) (-7.2799, -4.744) (-6.6328, -4.8971) (-6.3364, -5.1244) knots 0 0 0 1 2 2 2
  spline S209 degree 2 poles (-6.3364, -5.1244) (-6.035, -5.3516) (-5.709, -6.0432) (-5.709, -6.5965) knots 0 0 0 1 2 2 2
  line L202 (-3.234, -8.533) -> (-3.234, -3.1583)
  line L203 (-3.234, -3.1583) -> (-5.2792, -3.1583)
  line L204 (-5.2792, -3.1583) -> (-5.2792, -2.437)
  line L205 (-5.2792, -2.437) -> (-0.3787, -2.437)
  line L206 (-0.3787, -2.437) -> (-0.3787, -3.1583)
  line L207 (-0.3787, -3.1583) -> (-2.4239, -3.1583)
  line L208 (-2.4239, -3.1583) -> (-2.4239, -8.533)
  line L209 (-2.4239, -8.533) -> (-3.234, -8.533)
  line L210 (5.1443, -10.2176) -> (4.2057, -10.2176)
  spline S210 degree 2 poles (4.2057, -10.2176) (3.4943, -9.3728) (2.6792, -7.4808) (2.6792, -6.1914) knots 0 0 0 1 2 2 2
  spline S211 degree 2 poles (2.6792, -6.1914) (2.6792, -4.9317) (3.4844, -3.01) (4.2057, -2.1653) knots 0 0 0 1 2 2 2
  line L211 (4.2057, -2.1653) -> (5.1443, -2.1653)
  line L212 (5.1443, -2.1653) -> (5.1443, -2.2048)
  spline S212 degree 2 poles (5.1443, -2.2048) (4.8133, -2.5062) (4.2106, -3.2867) (3.9537, -3.8054) knots 0 0 0 1 2 2 2
  spline S213 degree 2 poles (3.9537, -3.8054) (3.7067, -4.3093) (3.4004, -5.5196) (3.4004, -6.1914) knots 0 0 0 1 2 2 2
  spline S214 degree 2 poles (3.4004, -6.1914) (3.4004, -6.8929) (3.6968, -8.0538) (3.9537, -8.5775) knots 0 0 0 1 2 2 2
  spline S215 degree 2 poles (3.9537, -8.5775) (4.2007, -9.0813) (4.8281, -9.8965) (5.1443, -10.178) knots 0 0 0 1 2 2 2
  line L213 (5.1443, -10.178) -> (5.1443, -10.2176)
  line L214 (9.8175, -6.4384) -> (9.0914, -6.4384)
  line L215 (9.0914, -6.4384) -> (9.0914, -8.533)
  line L216 (9.0914, -8.533) -> (8.3059, -8.533)
  line L217 (8.3059, -8.533) -> (8.3059, -6.4384)
  line L218 (8.3059, -6.4384) -> (5.6136, -6.4384)
  line L219 (5.6136, -6.4384) -> (5.6136, -5.5789)
  line L220 (5.6136, -5.5789) -> (8.3405, -2.437)
  line L221 (8.3405, -2.437) -> (9.0914, -2.437)
  line L222 (9.0914, -2.437) -> (9.0914, -5.7814)
  line L223 (9.0914, -5.7814) -> (9.8175, -5.7814)
  line L224 (9.8175, -5.7814) -> (9.8175, -6.4384)
  line L225 (8.3059, -5.7814) -> (8.3059, -3.4003)
  line L226 (8.3059, -3.4003) -> (6.2558, -5.7814)
  line L227 (6.2558, -5.7814) -> (8.3059, -5.7814)
  spline S216 degree 2 poles (14.2636, -5.485) (14.2636, -7.1251) (13.3101, -8.6614) (12.3172, -8.6614) knots 0 0 0 1 2 2 2
  spline S217 degree 2 poles (12.3172, -8.6614) (11.3094, -8.6614) (10.3659, -7.0955) (10.3659, -5.4899) knots 0 0 0 1 2 2 2
  spline S218 degree 2 poles (10.3659, -5.4899) (10.3659, -3.84) (11.3193, -2.3135) (12.3172, -2.3135) knots 0 0 0 1 2 2 2
  spline S219 degree 2 poles (12.3172, -2.3135) (13.32, -2.3135) (14.2636, -3.8943) (14.2636, -5.485) knots 0 0 0 1 2 2 2
  spline S220 degree 2 poles (13.2163, -7.3425) (13.3348, -7.0411) (13.4336, -6.1124) (13.4336, -5.485) knots 0 0 0 1 2 2 2
  spline S221 degree 2 poles (13.4336, -5.485) (13.4336, -4.8576) (13.3348, -3.9338) (13.2113, -3.6226) knots 0 0 0 1 2 2 2
  spline S222 degree 2 poles (13.2113, -3.6226) (13.0878, -3.3114) (12.6581, -2.9903) (12.3172, -2.9903) knots 0 0 0 1 2 2 2
  spline S223 degree 2 poles (12.3172, -2.9903) (11.9763, -2.9903) (11.5367, -3.3114) (11.4082, -3.6325) knots 0 0 0 1 2 2 2
  spline S224 degree 2 poles (11.4082, -3.6325) (11.2847, -3.9437) (11.1958, -4.8922) (11.1958, -5.4899) knots 0 0 0 1 2 2 2
  spline S225 degree 2 poles (11.1958, -5.4899) (11.1958, -6.1321) (11.2748, -6.9917) (11.4033, -7.3276) knots 0 0 0 1 2 2 2
  spline S226 degree 2 poles (11.4033, -7.3276) (11.5219, -7.6438) (11.9615, -7.9847) (12.3172, -7.9847) knots 0 0 0 1 2 2 2
  spline S227 degree 2 poles (12.3172, -7.9847) (12.6531, -7.9847) (13.0928, -7.6636) (13.2163, -7.3425) knots 0 0 0 1 2 2 2
  spline S228 degree 2 poles (18.838, -5.485) (18.838, -7.1251) (17.8846, -8.6614) (16.8917, -8.6614) knots 0 0 0 1 2 2 2
  spline S229 degree 2 poles (16.8917, -8.6614) (15.8839, -8.6614) (14.9404, -7.0955) (14.9404, -5.4899) knots 0 0 0 1 2 2 2
  spline S230 degree 2 poles (14.9404, -5.4899) (14.9404, -3.84) (15.8938, -2.3135) (16.8917, -2.3135) knots 0 0 0 1 2 2 2
  spline S231 degree 2 poles (16.8917, -2.3135) (17.8945, -2.3135) (18.838, -3.8943) (18.838, -5.485) knots 0 0 0 1 2 2 2
  spline S232 degree 2 poles (17.7908, -7.3425) (17.9093, -7.0411) (18.0081, -6.1124) (18.0081, -5.485) knots 0 0 0 1 2 2 2
  spline S233 degree 2 poles (18.0081, -5.485) (18.0081, -4.8576) (17.9093, -3.9338) (17.7858, -3.6226) knots 0 0 0 1 2 2 2
  spline S234 degree 2 poles (17.7858, -3.6226) (17.6623, -3.3114) (17.2325, -2.9903) (16.8917, -2.9903) knots 0 0 0 1 2 2 2
  spline S235 degree 2 poles (16.8917, -2.9903) (16.5508, -2.9903) (16.1111, -3.3114) (15.9827, -3.6325) knots 0 0 0 1 2 2 2
  spline S236 degree 2 poles (15.9827, -3.6325) (15.8592, -3.9437) (15.7703, -4.8922) (15.7703, -5.4899) knots 0 0 0 1 2 2 2
  spline S237 degree 2 poles (15.7703, -5.4899) (15.7703, -6.1321) (15.8493, -6.9917) (15.9778, -7.3276) knots 0 0 0 1 2 2 2
  spline S238 degree 2 poles (15.9778, -7.3276) (16.0963, -7.6438) (16.536, -7.9847) (16.8917, -7.9847) knots 0 0 0 1 2 2 2
  spline S239 degree 2 poles (16.8917, -7.9847) (17.2276, -7.9847) (17.6673, -7.6636) (17.7908, -7.3425) knots 0 0 0 1 2 2 2
  line L228 (20.5176, -8.533) -> (19.747, -8.533)
  line L229 (19.747, -8.533) -> (19.747, -2.1653)
  line L230 (19.747, -2.1653) -> (20.5176, -2.1653)
  line L231 (20.5176, -2.1653) -> (20.5176, -8.533)
  spline S240 degree 2 poles (25.4824, -6.1717) (25.4824, -7.2931) (24.3956, -8.6614) (23.5755, -8.6614) knots 0 0 0 1 2 2 2
  spline S241 degree 2 poles (23.5755, -8.6614) (23.205, -8.6614) (22.6764, -8.4787) (22.4196, -8.3206) knots 0 0 0 1 2 2 2
  line L232 (22.4196, -8.3206) -> (22.3702, -8.533)
  line L233 (22.3702, -8.533) -> (21.6489, -8.533)
  line L234 (21.6489, -8.533) -> (21.6489, -2.1653)
  line L235 (21.6489, -2.1653) -> (22.4196, -2.1653)
  line L236 (22.4196, -2.1653) -> (22.4196, -4.4377)
  spline S242 degree 2 poles (22.4196, -4.4377) (22.711, -4.1759) (23.3878, -3.8301) (23.8176, -3.8301) knots 0 0 0 1 2 2 2
  spline S243 degree 2 poles (23.8176, -3.8301) (24.5932, -3.8301) (25.4824, -5.07) (25.4824, -6.1717) knots 0 0 0 1 2 2 2
  spline S244 degree 2 poles (24.687, -6.231) (24.687, -5.4109) (24.1881, -4.5612) (23.6348, -4.5612) knots 0 0 0 1 2 2 2
  spline S245 degree 2 poles (23.6348, -4.5612) (23.3236, -4.5612) (22.6814, -4.8576) (22.4196, -5.0849) knots 0 0 0 1 2 2 2
  line L237 (22.4196, -5.0849) -> (22.4196, -7.708)
  spline S246 degree 2 poles (22.4196, -7.708) (22.711, -7.8513) (23.1606, -7.9698) (23.4273, -7.9698) knots 0 0 0 1 2 2 2
  spline S247 degree 2 poles (23.4273, -7.9698) (24.0152, -7.9698) (24.687, -7.135) (24.687, -6.231) knots 0 0 0 1 2 2 2
  spline S248 degree 2 poles (28.4958, -6.1914) (28.4958, -7.4561) (27.6856, -9.3728) (26.9693, -10.2176) knots 0 0 0 1 2 2 2
  line L238 (26.9693, -10.2176) -> (26.0307, -10.2176)
  line L239 (26.0307, -10.2176) -> (26.0307, -10.178)
  spline S249 degree 2 poles (26.0307, -10.178) (26.3469, -9.8965) (26.9842, -9.0715) (27.2213, -8.5775) knots 0 0 0 1 2 2 2
  spline S250 degree 2 poles (27.2213, -8.5775) (27.4782, -8.0489) (27.7746, -6.8732) (27.7746, -6.1914) knots 0 0 0 1 2 2 2
  spline S251 degree 2 poles (27.7746, -6.1914) (27.7746, -5.5146) (27.4732, -4.3142) (27.2213, -3.8054) knots 0 0 0 1 2 2 2
  spline S252 degree 2 poles (27.2213, -3.8054) (26.9743, -3.2966) (26.3419, -2.4864) (26.0307, -2.2048) knots 0 0 0 1 2 2 2
  line L240 (26.0307, -2.2048) -> (26.0307, -2.1653)
  line L241 (26.0307, -2.1653) -> (26.9693, -2.1653)
  spline S253 degree 2 poles (26.9693, -2.1653) (27.6807, -3.01) (28.4958, -4.9169) (28.4958, -6.1914) knots 0 0 0 1 2 2 2
  line L242 (-16.1942, -18.5699) -> (-19.1681, -18.5699)
  line L243 (-19.1681, -18.5699) -> (-19.1681, -17.9475)
  line L244 (-19.1681, -17.9475) -> (-18.0615, -17.9475)
  line L245 (-18.0615, -17.9475) -> (-18.0615, -13.8621)
  line L246 (-18.0615, -13.8621) -> (-19.1681, -13.8621)
  line L247 (-19.1681, -13.8621) -> (-19.1681, -13.3038)
  spline S254 degree 2 poles (-19.1681, -13.3038) (-18.5407, -13.3038) (-17.9479, -12.9482) (-17.9084, -12.4541) knots 0 0 0 1 2 2 2
  line L248 (-17.9084, -12.4541) -> (-17.2761, -12.4541)
  line L249 (-17.2761, -12.4541) -> (-17.2761, -17.9475)
  line L250 (-17.2761, -17.9475) -> (-16.1942, -17.9475)
  line L251 (-16.1942, -17.9475) -> (-16.1942, -18.5699)
  line L252 (-11.3134, -18.5699) -> (-15.0728, -18.5699)
  line L253 (-15.0728, -18.5699) -> (-15.0728, -17.7054)
  spline S255 degree 2 poles (-15.0728, -17.7054) (-14.6677, -17.325) (-13.9465, -16.6186) (-13.6007, -16.2382) knots 0 0 0 1 2 2 2
  spline S256 degree 2 poles (-13.6007, -16.2382) (-12.9041, -15.4725) (-12.3953, -14.5537) (-12.3953, -14.0646) knots 0 0 0 1 2 2 2
  spline S257 degree 2 poles (-12.3953, -14.0646) (-12.3953, -13.8077) (-12.5534, -13.4224) (-12.6967, -13.2989) knots 0 0 0 1 2 2 2
  spline S258 degree 2 poles (-12.6967, -13.2989) (-12.8399, -13.1754) (-13.2154, -13.0519) (-13.4426, -13.0519) knots 0 0 0 1 2 2 2
  spline S259 degree 2 poles (-13.4426, -13.0519) (-13.66, -13.0519) (-14.1046, -13.1606) (-14.3071, -13.2446) knots 0 0 0 1 2 2 2
  spline S260 degree 2 poles (-14.3071, -13.2446) (-14.48, -13.3137) (-14.8011, -13.5113) (-14.8999, -13.5805) knots 0 0 0 1 2 2 2
  line L254 (-14.8999, -13.5805) -> (-14.9444, -13.5805)
  line L255 (-14.9444, -13.5805) -> (-14.9444, -12.711)
  spline S261 degree 2 poles (-14.9444, -12.711) (-14.6924, -12.5875) (-13.7884, -12.3455) (-13.3833, -12.3455) knots 0 0 0 1 2 2 2
  spline S262 degree 2 poles (-13.3833, -12.3455) (-12.5287, -12.3455) (-11.5654, -13.2495) (-11.5654, -14.0201) knots 0 0 0 1 2 2 2
  spline S263 degree 2 poles (-11.5654, -14.0201) (-11.5654, -14.3808) (-11.7334, -14.9834) (-11.8816, -15.2403) knots 0 0 0 1 2 2 2
  spline S264 degree 2 poles (-11.8816, -15.2403) (-12.0298, -15.5071) (-12.4595, -16.0307) (-12.6967, -16.2827) knots 0 0 0 1 2 2 2
  spline S265 degree 2 poles (-12.6967, -16.2827) (-13.082, -16.7026) (-14.0255, -17.6017) (-14.3071, -17.8635) knots 0 0 0 1 2 2 2
  line L256 (-14.3071, -17.8635) -> (-11.3134, -17.8635)
  line L257 (-11.3134, -17.8635) -> (-11.3134, -18.5699)
  line L258 (-7.9641, -12.2022) -> (-10.3501, -19.8938)
  line L259 (-10.3501, -19.8938) -> (-11.0417, -19.8938)
  line L260 (-11.0417, -19.8938) -> (-8.6656, -12.2022)
  line L261 (-8.6656, -12.2022) -> (-7.9641, -12.2022)
  spline S266 degree 2 poles (-3.4983, -15.5219) (-3.4983, -17.162) (-4.4517, -18.6984) (-5.4447, -18.6984) knots 0 0 0 1 2 2 2
  spline S267 degree 2 poles (-5.4447, -18.6984) (-6.4525, -18.6984) (-7.396, -17.1324) (-7.396, -15.5268) knots 0 0 0 1 2 2 2
  spline S268 degree 2 poles (-7.396, -15.5268) (-7.396, -13.8769) (-6.4426, -12.3504) (-5.4447, -12.3504) knots 0 0 0 1 2 2 2
  spline S269 degree 2 poles (-5.4447, -12.3504) (-4.4419, -12.3504) (-3.4983, -13.9312) (-3.4983, -15.5219) knots 0 0 0 1 2 2 2
  spline S270 degree 2 poles (-4.5456, -17.3794) (-4.427, -17.078) (-4.3282, -16.1493) (-4.3282, -15.5219) knots 0 0 0 1 2 2 2
  spline S271 degree 2 poles (-4.3282, -15.5219) (-4.3282, -14.8945) (-4.427, -13.9707) (-4.5505, -13.6595) knots 0 0 0 1 2 2 2
  spline S272 degree 2 poles (-4.5505, -13.6595) (-4.674, -13.3483) (-5.1038, -13.0272) (-5.4447, -13.0272) knots 0 0 0 1 2 2 2
  spline S273 degree 2 poles (-5.4447, -13.0272) (-5.7856, -13.0272) (-6.2252, -13.3483) (-6.3537, -13.6694) knots 0 0 0 1 2 2 2
  spline S274 degree 2 poles (-6.3537, -13.6694) (-6.4772, -13.9806) (-6.5661, -14.9291) (-6.5661, -15.5268) knots 0 0 0 1 2 2 2
  spline S275 degree 2 poles (-6.5661, -15.5268) (-6.5661, -16.1691) (-6.487, -17.0286) (-6.3586, -17.3645) knots 0 0 0 1 2 2 2
  spline S276 degree 2 poles (-6.3586, -17.3645) (-6.24, -17.6807) (-5.8004, -18.0216) (-5.4447, -18.0216) knots 0 0 0 1 2 2 2
  spline S277 degree 2 poles (-5.4447, -18.0216) (-5.1088, -18.0216) (-4.6691, -17.7005) (-4.5456, -17.3794) knots 0 0 0 1 2 2 2
  spline S278 degree 2 poles (1.1354, -16.5939) (1.1354, -17.0632) (0.8242, -17.8585) (0.5624, -18.1253) knots 0 0 0 1 2 2 2
  spline S279 degree 2 poles (0.5624, -18.1253) (0.2907, -18.4069) (-0.391, -18.6984) (-0.8011, -18.6984) knots 0 0 0 1 2 2 2
  spline S280 degree 2 poles (-0.8011, -18.6984) (-1.2111, -18.6984) (-1.8879, -18.4217) (-2.1447, -18.1451) knots 0 0 0 1 2 2 2
  spline S281 degree 2 poles (-2.1447, -18.1451) (-2.4609, -17.8141) (-2.8166, -16.7026) (-2.8166, -15.8924) knots 0 0 0 1 2 2 2
  spline S282 degree 2 poles (-2.8166, -15.8924) (-2.8166, -15.0971) (-2.4906, -13.8176) (-2.1497, -13.3434) knots 0 0 0 1 2 2 2
  spline S283 degree 2 poles (-2.1497, -13.3434) (-1.8187, -12.879) (-0.7714, -12.3603) (-0.0848, -12.3603) knots 0 0 0 1 2 2 2